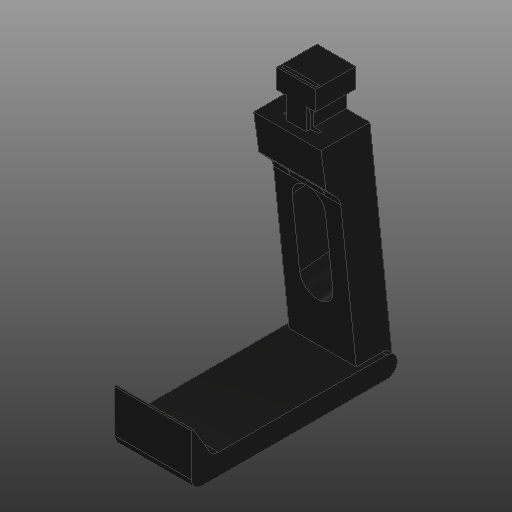
# Autodesk Inventor part: Lever1
Saved by Autodesk Inventor 2020 (Build 240168000, 168)
## iProperties
Created: 2019-12-28
Part Number: Lever1
Material: Generic
Document SubType Name: Modeling
Designer: Isaac Newcomb
Density: 1.06 g/cm^3
Appearance: Default
Mass: 2.49877 g
Surface Area: 21.9023 cm^2
Volume: 2.35733 cm^3
Project: Ice Keys
neckWidth: 2.800 mm
headWidth: 5.500 mm
headHeight: 2.800 mm
Author: Isaac Newcomb
Autodesk Inventor part; units mm, degrees
ref_plane "YZ Plane" through (0, 0, 0) normal (1, 0, 0) x (0, 1, 0)
ref_plane "XZ Plane" through (0, 0, 0) normal (0, 1, 0) x (-1, 0, 0)
ref_plane "Neck Start Plane" through (0, 0, -1.8245) normal (0, 0, 1) x (1, 0, 0)
sketch "Arm Profile" plane through (0, 0, 0) normal (1, 0, 0) x (0, 1, 0)
  line L0 (-2, -0.55) -> (-2, -7.55)
  line L1 (-2, -7.55) -> (-34.3125, -10.9462)
  line L2 (-34.3125, 18.625) -> (-26.7563, 18.625)
  line L3 (-26.692, 18.3928) -> (-31.3125, 15.625)
  arc A0 (-26.692, 18.3928) -> (-26.7563, 18.625) centre (-26.7563, 18.5) ccw
  line L4 (0, 0) -> (-30.5125, 0) construction
  line L5 (-30.5125, 0) -> (-31.3125, 0) construction
  line L6 (-2, -2.9554) -> (-10.1292, -3.3815)
  line L7 (-2, -2.5) -> (-9, -2.8669)
  line L8 (-9, -2.8669) -> (-7.3168, -1.2972)
  line L9 (-7.3168, -1.2972) -> (-2, -0.55)
  line L10 (-10.1292, -3.3815) -> (-31.3125, -5.6079)
  arc A1 (-10.1292, -3.3815) -> (-9, -2.8669) centre (-10.3336, -1.4368) ccw
  line L11 (-2, -2.5) -> (3.8762, -2.192)
  line L12 (3.8762, -2.192) -> (3.9, -2.6462)
  line L13 (3.9, -2.6462) -> (-2, -2.9554)
  line L14 (-31.3125, -5.6079) -> (-31.3125, 15.625)
  line L15 (-34.3125, -10.9462) -> (-34.3125, 18.625)
  line L16 (-31.3125, -5.6079) -> (-31.3125, -10.6309)
  line L17 (-24.5249, -9.9175) -> (-25.047, -4.9494)
  line L18 (-10.1292, -3.3815) -> (-9.607, -8.3495)
  point P0 (-7.4117, -1.3306)
  dimension "d0" = 0.125
  dimension "d1" = 26.7563
  dimension "d2" = 18.5
  dimension "d7" = 3
  dimension "d85" = 2
  dimension "neckDepth" = 7
  dimension "d119" = 30.5125
  dimension "d121" = 0.55
  dimension "d129" = 0.4548
  dimension "d132" = 8
  dimension "d136" = 145
  dimension "d137" = 7
  dimension "d138" = 5.9
  dimension "pincherArmThick" = 3
  dimension "d141" = 0.8
  dimension "d147" = 15
  dimension "d148" = 6
  dimension "d151" = 177
  dimension "d153" = 2.5
  constraints: 40 end point, 7 point on line, 4 perpendicular, 4 point on circle, 4 tangent, 3 collinear, 2 centre point, 2 horizontal, 2 parallel, 2 vertical, 1 coincident
  measures "d0" radius of A0
  measures "d1" horizontal distance of A0.centre point (0, 0)
  measures "d2" vertical distance of A0.centre point (0, 0)
  measures "d7" distance from line of L3.end L2
  measures "d85" distance from line of point (0, 0) L0
  measures "neckDepth" distance of L0.start L0.end
  measures "d119" distance of L4.start L4.end
  measures "d121" vertical distance of point (0, 0) L0.start
  measures "d129" distance between parallel lines of L6 L7
  measures "d132" angle of L4 L9
  measures "d136" angle of L9 L8
  measures "d137" distance from line of L0 L7.end
  measures "d138" distance from line of L0 L12.end
  measures "pincherArmThick" distance between parallel lines of L14 L15
  measures "d141" distance from line of L4.end L14
  measures "d147" distance between parallel lines of L17 L18
  measures "d148" angle of L4 L10
  measures "d151" angle of L10 L6
  measures "d153" vertical distance of L7.start point (0, 0)
extrude "Main Arm" add sketch "Arm Profile" along normal mid plane 9.6 contours L0 L7 L8 L9 | L0 L6 A1 L7 | L0 L1 L18 L6 | L18 L1 L17 L10 | L17 L1 L16 L10
extrude "Pincher" add sketch "Arm Profile" along normal mid plane 11 contours L16 L1 L15 L2 A0 L3 L14
sketch "Neck Sketch" plane through (0, 0, -1.8245) normal (0, 0, 1) x (1, 0, 0)
  line L0 (-1.4, -2) -> (-1.4, 1.1)
  line L1 (-2.75, 3.9) -> (2.75, 3.9)
  line L2 (1.4, 1.1) -> (1.4, -2)
  line L3 (0, -2) -> (0, 3.9) construction
  line L4 (-1.4, 1.1) -> (-2.75, 1.1)
  line L5 (-2.75, 1.1) -> (-2.75, 3.9)
  line L6 (2.75, 3.9) -> (2.75, 1.1)
  line L7 (2.75, 1.1) -> (1.4, 1.1)
  line L8 (1.4, -2) -> (-1.4, -2)
  point P0 (0, 0)
  dimension "neckWidth" = 2.8
  dimension "headWidth" = 5.5
  dimension "headHeight" = 2.8
  dimension "d91" = 2
  dimension "d103" = 1.1
  dimension "neckHeight" = 5.9
  constraints: 18 end point, 3 parallel, 3 perpendicular, 2 horizontal, 2 midpoint, 2 point on line, 2 vertical
  measures "neckWidth" distance of L2.end L0.start
  measures "headWidth" distance of L1.start L1.end
  measures "headHeight" vertical distance of L0.end L1.start
  measures "d91" distance from line of L8 point (0, 0)
  measures "d103" distance from line of point (0, 0) L7
  measures "neckHeight" distance between parallel lines of L1 L8
extrude "Neck" add sketch "Neck Sketch" against normal blind 5.7255
extrude "Spring Steel Slot" cut sketch "Arm Profile" along normal mid plane 4.9625 contours L11 L12 L13 L0 | L0 L6 A1 L7
extrude "Viewport" cut sketch "Arm Profile" along normal mid plane 4.7625 contours L18 L1 L17 L10
fillet "Fillet1" radius 1.5 5 edges at (-5.15, -31.3125, -10.6309) (5.15, -31.3125, -10.6309) (0, -34.3125, -10.9462) (0, -31.3125, 15.625) (0, -34.3125, 18.625)
fillet "Fillet2" radius 2.3813 4 edges at (-2.3813, -24.7859, -7.4334) (2.3813, -24.7859, -7.4334) (2.3813, -9.8681, -5.8655) (-2.3813, -9.8681, -5.8655)
equation "\"d2\" = hingeToPincherHoriz"
equation "\"spacing\" = 1"
equation "\"hingeToPincherHoriz\" = 18.5"
body "Solid1"
